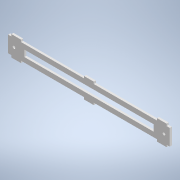
# Autodesk Inventor part: Base_Carril
Saved by Autodesk Inventor 2022 (Build 260153000, 153)
## iProperties
Created: 2022-01-30
Part Number: Base_Carril
Material: Generic
Document SubType Name: Modeling
Designer: katha
Density: 1 g/cm^3
Appearance: Default
Author: katha
Autodesk Inventor part; units mm, degrees
ref_plane "YZ Plane" through (0, 0, 0) normal (1, 0, 0) x (0, 1, 0)
ref_plane "XZ Plane" through (0, 0, 0) normal (0, 1, 0) x (-1, 0, 0)
ref_plane "XY Plane" through (0, 0, 0) normal (0, 0, 1) x (1, 0, 0)
sketch "Sketch1" plane through (0, 0, 0) normal (0, 0, 1) x (1, 0, 0)
  line L0 (-125, 12.5) -> (125, 12.5)
  line L1 (125, 12.5) -> (125, -12.5)
  line L2 (125, -12.5) -> (-125, -12.5)
  line L3 (-125, -12.5) -> (-125, 12.5)
  line L4 (-125, 12.5) -> (125, -12.5) construction
  line L5 (125, 12.5) -> (-125, -12.5) construction
  line L6 (100, -5) -> (-100, -5)
  line L7 (-100, -5) -> (-100, 5)
  line L8 (-100, 5) -> (100, 5)
  line L9 (100, 5) -> (100, -5)
  line L10 (100, -5) -> (-100, 5) construction
  line L11 (-100, -5) -> (100, 5) construction
  line L12 (-120, 12.5) -> (-120, 15.7)
  line L13 (-120, 15.7) -> (-105, 15.7)
  line L14 (-105, 15.7) -> (-105, 12.5)
  line L15 (-7.5, 12.5) -> (-7.5, 15.7)
  line L16 (-7.5, 15.7) -> (7.5, 15.7)
  line L17 (7.5, 15.7) -> (7.5, 12.5)
  line L18 (0, 0) -> (0, 12.5) construction
  line L19 (0, 0) -> (31.571, 0) construction
  line L20 (120, 12.5) -> (120, 15.7)
  line L21 (120, 15.7) -> (105, 15.7)
  line L22 (105, 15.7) -> (105, 12.5)
  line L23 (-120, -12.5) -> (-120, -15.7)
  line L24 (-120, -15.7) -> (-105, -15.7)
  line L25 (-105, -15.7) -> (-105, -12.5)
  line L26 (-7.5, -12.5) -> (-7.5, -15.7)
  line L27 (-7.5, -15.7) -> (7.5, -15.7)
  line L28 (7.5, -15.7) -> (7.5, -12.5)
  line L29 (120, -12.5) -> (120, -15.7)
  line L30 (120, -15.7) -> (105, -15.7)
  line L31 (105, -15.7) -> (105, -12.5)
  circle A0 centre (-116, 0) radius 2 projected
  circle A1 centre (-116, 0) radius 2
  circle A2 centre (116, 0) radius 2
  dimension "d0" = 250
  dimension "d1" = 25
  dimension "d6" = 200
  dimension "d7" = 10
  dimension "d10" = 3.2
  dimension "d11" = 15
  dimension "d12" = 5
  dimension "d13" = 3.2
  dimension "d14" = 15
  dimension "d15" = 7.5
  constraints: 64 end point, 17 symmetric about line, 7 perpendicular, 5 midpoint, 4 parallel, 4 point on line, 3 horizontal, 2 centre point, 1 coincident, 1 concentric, 1 vertical, 1 other
  measures "d0" distance of L1.end L2.end
  measures "d1" distance of L0.end L1.end
  measures "d6" distance of L7.end L8.end
  measures "d7" distance of L6.end L7.end
  measures "d10" distance of L12.start L12.end
  measures "d11" distance of L12.end L13.end
  measures "d12" distance between parallel lines of L12 L3
  measures "d13" distance of L15.start L15.end
  measures "d14" distance of L15.end L16.end
  measures "d15" distance from line of L15 L18.start
extrude "Extrusion4" add sketch "Sketch1" along normal blind 3.2
body "Solid3"
